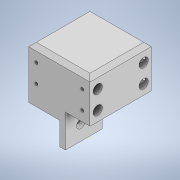
# Autodesk Inventor part: (FINAL)CORNER
Saved by Autodesk Inventor 2022 (Build 260153000, 153)
## iProperties
Created: 2022-11-16
Part Number: (FINAL)CORNER
Material: Generic
Document SubType Name: Modeling
Designer: matia
Density: 1 g/cm^3
Appearance: Default
Author: matia
Autodesk Inventor part; units mm, degrees
ref_plane "YZ Plane" through (0, 0, 0) normal (1, 0, 0) x (0, 1, 0)
ref_plane "XZ Plane" through (0, 0, 0) normal (0, 1, 0) x (-1, 0, 0)
ref_plane "XY Plane" through (0, 0, 0) normal (0, 0, 1) x (1, 0, 0)
sketch "Sketch1" plane through (0, 0, 0) normal (0, 1, 0) x (-1, 0, 0)
  line L0 (25.4, 25.4) -> (-25.4, 25.4)
  line L1 (-25.4, 25.4) -> (-25.4, -25.4)
  line L2 (-25.4, -25.4) -> (25.4, -25.4)
  line L3 (25.4, -25.4) -> (25.4, 25.4)
  line L4 (25.4, 25.4) -> (-25.4, -25.4) construction
  line L5 (-25.4, 25.4) -> (25.4, -25.4) construction
  point P0 (0, 0)
  dimension "d0" = 50.8
  dimension "d1" = 50.8
  constraints: 12 end point, 2 midpoint, 2 parallel, 1 horizontal, 1 perpendicular
  measures "d0" distance of L2.end L1.end
  measures "d1" distance of L1.end L0.end
extrude "Extrusion1" add sketch "Sketch1" along normal mid plane 38.1
sketch "Sketch2" plane through (25.4, -19.05, -25.4) normal (1, 0, 0) x (0, 0, -1)
  line L0 (-50.8, 38.1) -> (0, 38.1) projected
  line L1 (-50.8, 38.1) -> (-44.45, 38.1)
  line L2 (-44.45, 38.1) -> (-44.45, 0)
  line L3 (-50.8, 0) -> (0, 0) projected
  line L4 (0, 0) -> (0, 38.1) projected
  line L5 (0, 38.1) -> (-6.35, 38.1)
  line L6 (-6.35, 38.1) -> (-6.35, 0)
  line L7 (-6.35, 0) -> (0, 0)
  line L8 (0, 0) -> (0, 11.43)
  line L9 (0, 11.43) -> (-50.8, 11.43)
  line L10 (-50.8, 0) -> (-50.8, 38.1) projected
  line L11 (-50.8, 38.1) -> (-50.8, 26.67)
  line L12 (-50.8, 26.67) -> (0, 26.67)
  circle A0 centre (-44.45, 26.67) radius 3.81
  circle A1 centre (-44.45, 11.43) radius 3.81
  circle A2 centre (-6.35, 26.67) radius 3.81
  circle A3 centre (-6.35, 11.43) radius 3.81
  point P0 (-25.4, 19.05)
  dimension "d4" = 6.35
  dimension "d5" = 6.35
  dimension "d6" = 11.43
  dimension "d7" = 11.43
  dimension "d8" = 7.62
  dimension "d9" = 7.62
  dimension "d10" = 7.62
  dimension "d11" = 7.62
  constraints: 18 end point, 13 point on line, 7 perpendicular, 4 centre point
  measures "d4" distance of L0.start L1.end
  measures "d5" distance of L0.end L5.end
  measures "d6" distance of L7.end L8.end
  measures "d7" distance of L0.start L11.end
  measures "d8" diameter of A0
  measures "d9" diameter of A1
  measures "d10" diameter of A2
  measures "d11" diameter of A3
sketch "Sketch3" plane through (25.4, 19.05, -25.4) normal (0, 0, -1) x (-1, 0, 0)
  line L0 (0, 0) -> (50.8, 0) projected
  line L1 (0, 0) -> (6.35, 0)
  line L2 (50.8, -38.1) -> (0, -38.1) projected
  line L3 (50.8, -38.1) -> (50.8, 0) projected
  line L4 (50.8, -38.1) -> (44.45, -38.1)
  line L5 (44.45, 0) -> (44.45, -7.62)
  line L6 (48.26, -11.43) -> (50.8, -11.43)
  line L7 (0, -38.1) -> (0, 0) projected
  line L8 (6.35, -38.1) -> (6.35, -30.48)
  line L9 (6.35, -26.67) -> (0, -26.67)
  circle A0 centre (6.35, -11.43) radius 3.81
  circle A1 centre (6.35, -26.67) radius 3.81
  circle A2 centre (44.45, -11.43) radius 3.81
  circle A3 centre (44.45, -26.67) radius 3.81
  line L10 (2.54, -11.43) -> (0, -11.43)
  line L11 (6.35, 0) -> (6.35, -7.62)
  line L12 (6.35, -15.24) -> (6.35, -22.86)
  line L13 (6.35, -30.48) -> (6.35, -38.1)
  line L14 (0, -26.67) -> (2.54, -26.67)
  line L15 (10.16, -26.67) -> (40.64, -26.67)
  line L16 (48.26, -26.67) -> (50.8, -26.67)
  line L17 (44.45, -38.1) -> (44.45, -30.48)
  line L18 (50.8, -11.43) -> (44.45, -11.43)
  line L19 (40.64, -11.43) -> (10.16, -11.43)
  line L20 (44.45, -22.86) -> (44.45, -15.24)
  line L21 (44.45, -7.62) -> (44.45, 0)
  point P0 (25.4, -19.05)
  dimension "d12" = 6.35
  dimension "d13" = 6.35
  dimension "d14" = 11.43
  dimension "d15" = 11.43
  dimension "d16" = 7.62
  dimension "d17" = 7.62
  dimension "d18" = 7.62
  dimension "d19" = 7.62
  constraints: 36 end point, 16 point on circle, 10 perpendicular, 6 point on line, 4 centre point, 2 coincident, 1 horizontal
  measures "d12" distance of L0.start L1.end
  measures "d13" distance of L2.start L4.end
  measures "d14" distance of L5.start L18.end
  measures "d15" distance of L9.start L8.start
  measures "d16" diameter of A0
  measures "d17" diameter of A1
  measures "d18" diameter of A2
  measures "d19" diameter of A3
extrude "Extrusion2" cut sketch "Sketch3" against normal blind 38.1 contours A0 | A2 | A1 | A3
extrude "Extrusion3" cut sketch "Sketch2" against normal blind 38.1 contours A0 L12 L2 | L2 L12 A0 | L12 L2 A0 | A2 L12 L6 | L6 L12 A2 | L12 A0 L2 | A1 L2 L9 | L9 L2 A1 | L12 A2 L6 | L6 A2 L12 | L9 A1 L2 | L2 A1 L9 | A3 L6 L9 | L9 L6 A3 | L6 L9 A3 | L9 L6 A3
sketch "Sketch4" plane through (-12.7, 7.62, 19.05) normal (1, 0, 0) x (0, 0, -1)
  circle A0 centre (0, 0) radius 3.5687
  circle A1 centre (0, 0) radius 0.8623
  point P0 (19.05, -7.62)
  dimension "d24" = 7.1374
  constraints: 2 centre point, 1 coincident
  measures "d24" diameter of A0
hole "Hole1" at (-12.7, 7.62, 19.05) direction (-1, 0, 0) diameter 2.4867 end through all thread size "5-40 UNC" class "2B" standard "ANSI Unified Screw Threads"
mirror "Mirror1" about plane through (0, 0, 0) normal (0, 1, 0) of "Hole1", "Extrusion3"
mirror "Mirror2" about plane through (0, 0, 0) normal (0, 0, 1) of "Hole1", "Extrusion3", "Mirror1"
sketch "Sketch5" plane through (19.05, 7.62, 12.7) normal (0, 0, -1) x (-1, 0, 0)
  circle A0 centre (0, 0) radius 3.5687
  point P0 (19.05, -7.62)
  dimension "d35" = 7.1374
  constraints: 1 centre point
  measures "d35" diameter of A0
hole "Hole2" at (19.05, 7.62, 12.7) direction (0, 0, 1) diameter 2.4867 end through all thread size "5-40 UNC" class "2B" standard "ANSI Unified Screw Threads"
mirror "Mirror3" about plane through (0, 0, 0) normal (0, 1, 0) of "Hole2", "Extrusion2"
sketch "Sketch6" plane through (-19.05, 7.62, 12.7) normal (0, 0, -1) x (-1, 0, 0)
  circle A0 centre (0, 0) radius 3.5687
  circle A1 centre (0, -15.1755) radius 3.5687
  point P0 (-19.05, -7.62)
  dimension "d46" = 7.1374
  dimension "d47" = 7.1374
  constraints: 2 centre point
  measures "d46" diameter of A0
  measures "d47" diameter of A1
hole "Hole3" at (-19.05, 7.62, 12.7) direction (0, 0, 1) diameter 2.4867 end through all thread size "5-40 UNC" class "2B" standard "ANSI Unified Screw Threads"
sketch "Sketch7" plane through (-19.05, -7.62, 12.7) normal (0, 0, -1) x (-1, 0, 0)
  circle A0 centre (0, 0) radius 3.5687
  point P0 (-19.05, 7.62)
  dimension "d55" = 7.1374
  constraints: 1 centre point
  measures "d55" diameter of A0
hole "Hole4" at (-19.05, -7.62, 12.7) direction (0, 0, 1) diameter 2.4867 end through all thread size "5-40 UNC" class "2B" standard "ANSI Unified Screw Threads"
sketch "Sketch8" plane through (0, -19.05, 0) normal (0, -1, 0) x (1, 0, 0)
  line L0 (-25.4, -25.4) -> (-25.4, 25.4) projected
  line L1 (-25.4, 0) -> (-25.4, -5.08)
  line L2 (-25.4, -5.08) -> (0, -5.08)
  line L3 (0, -5.08) -> (5.08, -5.08)
  line L4 (5.08, -5.08) -> (5.08, 0)
  line L5 (5.08, 0) -> (5.08, 25.4)
  line L6 (25.4, 25.4) -> (-25.4, 25.4) projected
  line L7 (0, 25.4) -> (5.08, 25.4)
  line L8 (0, 25.4) -> (0, 0)
  line L9 (0, 0) -> (-25.4, 0)
  line L10 (-22.86, -25.4) -> (-22.86, 12.7) projected
  point P0 (-22.86, 0)
  point P1 (-22.86, -5.08)
  dimension "d66" = 5.08
  dimension "d67" = 5.08
  constraints: 16 end point, 4 perpendicular, 4 point on line, 1 midpoint, 1 vertical
  measures "d66" distance of L1.start L1.end
  measures "d67" distance of L2.end L3.end
extrude "Extrusion4" add sketch "Sketch8" along normal blind 30.48 contours L10 L9 L8 L6 L5 L4 L3 L2
sketch "Sketch9" plane through (0, -19.05, 0) normal (0, -1, 0) x (1, 0, 0)
  line L0 (0, 0) -> (0, 25.4) projected
  line L1 (-25.4, 25.4) -> (-25.4, -25.4) projected
  line L2 (0, 0) -> (-25.4, 0)
  line L3 (-25.4, 0) -> (-25.4, 25.4)
  line L4 (-25.4, 25.4) -> (0, 25.4)
  line L5 (0, 25.4) -> (0, 0)
  line L6 (-22.86, 0) -> (-22.86, -5.08) projected
  line L7 (-25.4, 0) -> (-22.86, -5.08)
  line L8 (-22.86, -5.08) -> (-25.4, -5.08)
  line L9 (-22.86, 0) -> (0, 0) projected
  line L10 (-25.4, 0) -> (-22.86, 0)
  line L11 (-22.86, 0) -> (-22.86, -5.08)
  constraints: 16 end point, 3 perpendicular, 2 horizontal, 2 parallel, 1 point on line
extrude "Extrusion5" add sketch "Sketch9" along normal blind 30.48 contours L6 L7 L2 | L7 L8 L1
sketch "Sketch10" plane through (0, -19.05, 0) normal (0, -1, 0) x (1, 0, 0)
  line L0 (0, 25.4) -> (0, 0) projected
  line L1 (0, 25.4) -> (-25.4, 25.4) projected
  line L2 (0, 0) -> (-25.4, 0)
  line L3 (-25.4, 0) -> (-25.4, 25.4)
  line L4 (-25.4, 25.4) -> (0, 25.4)
  line L5 (0, 25.4) -> (0, 0)
  constraints: 8 end point, 2 parallel, 1 horizontal, 1 perpendicular
extrude "Extrusion6" add sketch "Sketch10" along normal blind 5.08
sketch "Sketch11" plane through (5.08, -19.05, -5.08) normal (0, 0, -1) x (-1, 0, 0)
  line L0 (5.08, -5.08) -> (30.48, -5.08) projected
  line L1 (5.08, -5.08) -> (5.08, -30.48) projected
  line L2 (30.48, -5.08) -> (5.08, -5.08)
  line L3 (5.08, -5.08) -> (17.78, -5.08)
  line L4 (17.78, -5.08) -> (17.78, -11.43)
  circle A0 centre (17.78, -11.43) radius 2.2835
  point P0 (5.08, 19.05)
  dimension "d74" = 6.35
  constraints: 6 end point, 2 perpendicular, 1 centre point, 1 coincident, 1 midpoint
  measures "d74" distance of L3.end L4.end
sketch "Sketch12" plane through (5.08, -19.05, 25.4) normal (1, 0, 0) x (0, 0, -1)
  line L0 (0, -5.08) -> (25.4, -5.08) projected
  line L1 (25.4, -5.08) -> (0, -5.08)
  line L2 (0, -5.08) -> (12.7, -5.08)
  line L3 (12.7, -5.08) -> (12.7, -11.43)
  circle A0 centre (12.7, -11.43) radius 2.3644
  point P0 (25.4, 19.05)
  dimension "d85" = 6.35
  constraints: 6 end point, 1 centre point, 1 coincident, 1 collinear, 1 midpoint, 1 perpendicular
  measures "d85" distance of L2.end L3.end
chamfer "Chamfer6" distance 3.175 angle 45 8 edges at (25.4, 19.05, 0) (0, 19.05, -25.4) (-25.4, 19.05, 0) (0, 19.05, 25.4) (25.4, -19.05, 0) (0, -19.05, -25.4) (-25.4, -19.05, -15.24) (15.24, -19.05, 25.4)
sketch "Sketch13" plane through (-12.7, -7.62, 19.05) normal (1, 0, 0) x (0, 0, -1)
  circle A0 centre (0, 0) radius 3.5687
  point P0 (19.05, 7.62)
  dimension "d99" = 7.1374
  constraints: 1 centre point
  measures "d99" diameter of A0
sketch "Sketch14" plane through (-12.7, 7.62, 19.05) normal (1, 0, 0) x (0, 0, -1)
  point P0 (19.05, -7.62)
chamfer "Chamfer7" distance 2.3241 angle 45 1 edges at (-12.7, 7.62, 20.2933)
chamfer "Chamfer8" distance 2.3241 angle 45 3 edges at (-12.7, -7.62, 20.2933) (-12.7, -7.62, -20.2933) (-12.7, 7.62, -20.2933)
chamfer "Chamfer9" distance 2.3241 angle 45 4 edges at (19.05, 6.3767, 12.7) (19.05, -6.3767, 12.7) (-19.05, 6.3767, 12.7) (-19.05, -8.8633, 12.7)
sketch "Sketch15" plane through (0, -24.13, 0) normal (0, -1, 0) x (1, 0, 0)
  line L0 (0, 25.4) -> (0, 0) projected
  line L1 (0, 0) -> (0, 12.7)
  line L2 (0, 12.7) -> (0, 0)
  line L3 (0, 0) -> (-25.4, 0) projected
  line L4 (0, 0) -> (-12.7, 0)
  line L5 (-12.7, 0) -> (-12.7, 12.7)
  circle A0 centre (-12.7, 12.7) radius 12.7
  dimension "d112" = 12.7
  dimension "d113" = 12.7
  dimension "d114" = 12.7
  constraints: 8 end point, 2 midpoint, 1 coincident, 1 collinear, 1 perpendicular, 3 other
  measures "d112" distance of L0.end L1.end
  measures "d113" distance of L0.end L4.end
  measures "d114" distance of L4.end L5.end
extrude "Extrusion7" add sketch "Sketch15" along normal blind 25.4 contours L0 L3 A0
ref_plane "Work Plane1" through (-12.7, -30.48, 0) normal (0, 0, -1) x (-1, 0, 0)
sketch "Sketch16" plane through (-12.7, -30.48, 0) normal (0, 0, -1) x (-1, 0, 0)
  arc A0 (0, 1.2433) -> (0, -1.2433) centre (0, 0) ccw projected
  circle A1 centre (0, 0) radius 1.2433
  point P0 (-12.7, 30.48)
  constraints: 1 centre point, 1 coincident
hole "Hole7" at (5.08, -30.48, 12.7) direction (-1, 0, 0) diameter 2.4867 end through all thread size "5-40 UNC" class "2B" standard "ANSI Unified Screw Threads"
hole "Hole8" at (-12.7, -30.48, -5.08) direction (0, 0, 1) diameter 2.4867 end through all thread size "5-40 UNC" class "2B" standard "ANSI Unified Screw Threads"
chamfer "Chamfer11" distance 2.3241 angle 45 1 edges at (-12.7, -31.7233, -5.08)
chamfer "Chamfer12" distance 2.3241 angle 45 1 edges at (5.08, -30.48, 13.9433)
sketch "Sketch17" plane through (0, -49.53, 0) normal (0, -1, 0) x (1, 0, 0)
  line L0 (-25.4, -25.4) -> (-25.4, 25.4) projected
  line L1 (-25.4, 0) -> (-25.4, -0.254)
  line L2 (0, 0) -> (0, -0.254)
  line L3 (0, -0.254) -> (-25.4, -0.254)
  line L4 (5.08, 25.4) -> (0, 25.4) projected
  line L5 (0, 25.4) -> (0.254, 25.4)
  line L6 (0, 25.4) -> (-25.4, 25.4) projected
  line L7 (0.254, 25.4) -> (0.254, -0.254)
  line L8 (0.254, -0.254) -> (0.254, -0.254)
  line L9 (0.254, -0.254) -> (0, -0.254)
  arc A0 (-12.7, 0) -> (0, 12.7) centre (-12.7, 12.7) ccw projected
  circle A1 centre (-12.7, 12.7) radius 12.954
  point P0 (-12.7, -0.254)
  point P1 (0.254, 12.7)
  point P2 (-15.2527, 25.4)
  point P3 (-25.4, 15.2527)
  dimension "d137" = 0.254
  dimension "d138" = 0.254
  constraints: 14 end point, 3 perpendicular, 2 point on line, 1 centre point, 1 coincident, 1 collinear, 1 midpoint, 1 vertical
  measures "d137" distance of L1.start L1.end
  measures "d138" distance of L4.end L5.end
sketch "Sketch18" plane through (0, -49.53, 0) normal (0, -1, 0) x (1, 0, 0)
  point P0 (0, 0)
extrude "Extrusion8" cut sketch "Sketch17" against normal blind 25.4 contours L0 A1 L3 | A1 L0 L6 | A1 L6 L4 L7 picked at (-18.8184, 12.7418)
sketch "Sketch19" plane through (0, -49.53, 0) normal (0, -1, 0) x (1, 0, 0)
  point P0 (0, 0)
sketch "Sketch20" plane through (0, -49.53, 0) normal (0, -1, 0) x (1, 0, 0)
  point P0 (0, 0)
sketch "Sketch21" plane through (0, -49.53, 0) normal (0, -1, 0) x (1, 0, 0)
  line L0 (5.08, -5.08) -> (5.08, 25.4) projected
  line L1 (-25.4, 25.4) -> (25.4, 25.4) projected
  line L2 (5.08, -5.08) -> (-25.4, -5.08)
  line L3 (-25.4, -5.08) -> (-25.4, 25.4)
  line L4 (-25.4, 25.4) -> (5.08, 25.4)
  line L5 (5.08, 25.4) -> (5.08, -5.08)
  point P0 (0, 0)
  constraints: 8 end point, 2 parallel, 1 horizontal, 1 perpendicular
extrude "Extrusion9" cut sketch "Sketch21" against normal blind 6.35
body "Solid1"
